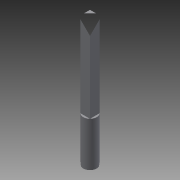
# Autodesk Inventor part: shaft_adapter
Saved by Autodesk Inventor 2015 (Build 190159000, 159)
## iProperties
Created: 2015-12-08
Part Number: shaft_adapter
Material: Generic
Document SubType Name: Modeling
Designer: boztalay
Density: 1 g/cm^3
Appearance: Default
Author: boztalay
Autodesk Inventor part; units mm, degrees
ref_plane "YZ Plane" through (0, 0, 0) normal (1, 0, 0) x (0, 1, 0)
ref_plane "XZ Plane" through (0, 0, 0) normal (0, 1, 0) x (-1, 0, 0)
ref_plane "XY Plane" through (0, 0, 0) normal (0, 0, 1) x (1, 0, 0)
sketch "Sketch1" plane through (0, 0, 0) normal (0, 1, 0) x (-1, 0, 0)
  circle A0 centre (0, 0) radius 2.032
  dimension "d0" = 4.064
  constraints: 1 centre point, 1 coincident
  measures "d0" diameter of A0
extrude "Extrusion1" add sketch "Sketch1" along normal blind 13.335
sketch "Sketch2" plane through (0, 13.335, 0) normal (0, 1, 0) x (1, 0, 0)
  circle A0 centre (0, 0) radius 2.032 projected
  line L0 (1.4368, 1.4368) -> (-1.4368, 1.4368)
  line L1 (-1.4368, 1.4368) -> (-1.4368, -1.4368)
  line L2 (-1.4368, -1.4368) -> (1.4368, -1.4368)
  line L3 (1.4368, -1.4368) -> (1.4368, 1.4368)
  line L4 (1.4368, 1.4368) -> (-1.4368, -1.4368) construction
  line L5 (-1.4368, 1.4368) -> (1.4368, -1.4368) construction
  constraints: 12 end point, 2 midpoint, 2 parallel, 2 perpendicular, 1 horizontal, 2 other
extrude "Extrusion2" add sketch "Sketch2" along normal blind 25.4 contours L3 L2 L1 L0
hole "Hole2" at (0, 0, 0) direction (0, 1, 0) diameter 2.54 depth 15.875
body "Solid1"
